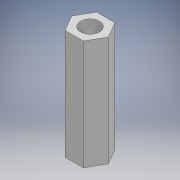
# Autodesk Inventor part: spacer
Saved by Autodesk Inventor 2017.2 (Build 212233000, 233)
## iProperties
Created: 2017-09-05
Part Number: spacer
Material: Generic
Document SubType Name: Modeling
Designer: Nic
Density: 1 g/cm^3
Appearance: Default
Author: Nic
Autodesk Inventor part; units mm, degrees
ref_plane "YZ Plane" through (0, 0, 0) normal (1, 0, 0) x (0, 1, 0)
ref_plane "XZ Plane" through (0, 0, 0) normal (0, 1, 0) x (-1, 0, 0)
ref_plane "XY Plane" through (0, 0, 0) normal (0, 0, 1) x (1, 0, 0)
sketch "Sketch1" plane through (0, 0, 0) normal (0, 0, 1) x (1, 0, 0)
  line L0 (-1.3279, 2.3) -> (1.3279, 2.3)
  line L1 (0, 2.3) -> (0, 0) construction
  circle A0 centre (0, 0) radius 2.3 construction
  line L2 (-2.656, 0) -> (-1.3279, 2.3)
  line L3 (-1.9919, 1.15) -> (0, 0) construction
  line L4 (-1.3282, -2.3001) -> (-2.656, 0)
  line L5 (-1.9919, -1.15) -> (0, 0) construction
  line L6 (1.3277, -2.3001) -> (-1.3282, -2.3001)
  line L7 (0, -2.3) -> (0, 0) construction
  line L8 (2.6557, -0.0001) -> (1.3277, -2.3001)
  line L9 (1.9919, -1.15) -> (0, 0) construction
  line L10 (1.3279, 2.3) -> (2.6557, -0.0001)
  line L11 (1.9919, 1.15) -> (0, 0) construction
  circle A1 centre (0, 0) radius 1.375
  point P0 (-2.656, 0)
  point P1 (2.6557, -0.0001)
  point P2 (-2.656, 0)
  dimension "d8" = 120
  dimension "d9" = 120.003
  dimension "d11" = 4.6
  dimension "d0" = 2.3
  dimension "d13" = 2.75
  constraints: 14 end point, 7 horizontal, 2 coincident, 1 centre point, 1 midpoint, 1 point on line, 1 vertical, 1 vertical alignment, 22 other
  measures "d0" distance of L1.start L1.end
  measures "d13" diameter of A1
extrude "Extrusion1" add sketch "Sketch1" along normal blind 16
body "Solid1"
